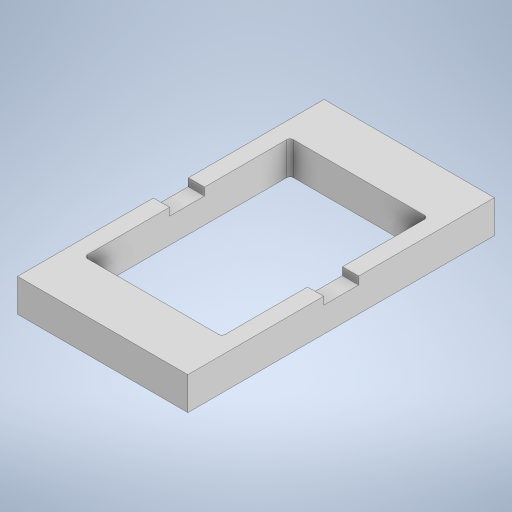
# Autodesk Inventor part: Cutter-bed
Saved by Autodesk Inventor 2024.1 (Build 281209000, 209)
## iProperties
Created: 2023-11-07
Part Number: Cutter-bed
Material: Generic
Document SubType Name: Modeling
Designer: katch
Density: 1 g/cm^3
Appearance: Default
Author: katch
Autodesk Inventor part; units mm, degrees
ref_plane "YZ Plane" through (0, 0, 0) normal (1, 0, 0) x (0, 1, 0)
ref_plane "XZ Plane" through (0, 0, 0) normal (0, 1, 0) x (-1, 0, 0)
ref_plane "XY Plane" through (0, 0, 0) normal (0, 0, 1) x (1, 0, 0)
sketch "Sketch1" plane through (0, 0, 0) normal (0, 1, 0) x (-1, 0, 0)
  line L0 (50, 90) -> (-50, 90)
  line L1 (-50, 90) -> (-50, -90)
  line L2 (-50, -90) -> (50, -90)
  line L3 (50, -90) -> (50, 90)
  point P0 (0, 0)
  dimension "d0" = 100
  dimension "d1" = 180
  constraints: 8 end point, 2 parallel, 1 horizontal, 1 perpendicular
  measures "d0" distance of L2.end L1.end
  measures "d1" distance of L1.end L0.end
extrude "Extrusion1" add sketch "Sketch1" along normal blind 19.3
sketch "Sketch2" plane through (0, 19.3, 0) normal (0, 1, 0) x (1, 0, 0)
  line L0 (40.5, -60.5) -> (-40.5, -60.5)
  line L1 (-40.5, -60.5) -> (-40.5, 60.5)
  line L2 (-40.5, 60.5) -> (40.5, 60.5)
  line L3 (40.5, 60.5) -> (40.5, -60.5)
  line L4 (40.5, -60.5) -> (-40.5, 60.5) construction
  line L5 (-40.5, -60.5) -> (40.5, 60.5) construction
  point P0 (0, 0)
  dimension "d4" = 81
  dimension "d5" = 121
  constraints: 12 end point, 2 midpoint, 2 parallel, 1 horizontal, 1 perpendicular
  measures "d4" distance of L1.end L2.end
  measures "d5" distance of L0.end L1.end
extrude "Extrusion2" cut sketch "Sketch2" against normal blind 19.3
fillet "Fillet1" radius 2 4 edges at (-40.5, 9.65, -60.5) (-40.5, 9.65, 60.5) (40.5, 9.65, 60.5) (40.5, 9.65, -60.5)
sketch "Sketch3" plane through (0, 19.3, 0) normal (0, 1, 0) x (1, 0, 0)
  line L0 (-50, 90) -> (-50, -90) projected
  line L1 (-40.5, -58.5) -> (-40.5, 58.5) projected
  line L2 (-50, 10.25) -> (-40.5, 10.25)
  line L3 (-40.5, 10.25) -> (-40.5, -10.25)
  line L4 (-40.5, -10.25) -> (-50, -10.25)
  line L5 (-50, -10.25) -> (-50, 10.25)
  line L6 (40.5, 58.5) -> (40.5, -58.5) projected
  line L7 (50, -90) -> (50, 90) projected
  line L8 (40.5, 10.25) -> (50, 10.25)
  line L9 (50, 10.25) -> (50, -10.25)
  line L10 (50, -10.25) -> (40.5, -10.25)
  line L11 (40.5, -10.25) -> (40.5, 10.25)
  point P0 (0, 0)
  dimension "d9" = 20.5
  constraints: 16 end point, 4 parallel, 4 point on line, 2 horizontal, 2 perpendicular
  measures "d9" distance of L2.end L3.end
extrude "Extrusion3" cut sketch "Sketch3" against normal blind 4.5
body "Solid1"
